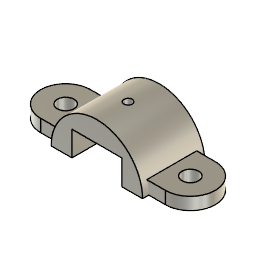
3.2 EDM (Autodesk Fusion 360 design; units mm, degrees)
Autodesk Fusion 360 part; units mm, degrees
sketch "Sketch1" plane through (0, 0, 0) normal (0, 1, 0) x (1, 0, 0)
  line L0 (-60, 0) -> (-60, -60)
  line L1 (-60, -60) -> (60, -60)
  line L2 (60, -60) -> (60, 0)
  line L3 (60, 60) -> (-60, -60) construction
  line L4 (-60, 60) -> (60, -60) construction
  arc A0 (-110, 0) -> (110, 0) centre (0, 0) ccw
  line L5 (-110, 0) -> (-60, 0)
  line L6 (60, 0) -> (110, 0)
  dimension "d1" = 220
  dimension "d2" = 120
  dimension "d3" = 120
  constraint coincident A0.centre origin
  constraint horizontal L5
  constraint parallel L0 L2
  constraint coincident L3 A0.centre
  constraint coincident L4 A0.centre
  constraint coincident L2.end L5
  constraint collinear L5 L6
  measures "d1" diameter of A0
  measures "d2" distance of L0.end L1.end
  measures "d3" distance of L4.start L0.end
extrude "Extrude1" add sketch "Sketch1" along normal mid plane 150 makes body 1
sketch "Sketch2" plane through (0, 0, 0) normal (0, 0, 1) x (1, 0, 0)
  circle A0 centre (0, 0) radius 10
  dimension "d6" = 20
  constraint coincident A0.centre origin
  measures "d6" diameter of A0
extrude "Extrude2" cut sketch "Sketch2" along normal blind 140 bodies 1
sketch "Sketch3" plane through (0, 0, 0) normal (0, 0, 1) x (1, 0, 0)
  line L0 (0, 0) -> (-153.6807, 0)
  line L1 (-153.6807, 0) -> (150, 0)
  line L2 (0, 120) -> (0, -100)
  circle A0 centre (150, 0) radius 20
  line L3 (150, 60) -> (105, 60)
  line L4 (105, 60) -> (105, 76.2902)
  line L5 (150, -60) -> (105, -60)
  line L6 (105, -60) -> (105, -75.5566)
  arc A1 (150, -60) -> (150, 60) centre (150, 0) ccw
  line L7 (105, 60) -> (105, -60)
  dimension "d9" = 120
  dimension "d10" = 40
  dimension "d11" = 150
  constraint coincident L0.start origin
  constraint horizontal L0
  constraint parallel L0 L1
  constraint perpendicular L1 L2
  constraint coincident L1.end A0.centre
  constraint concentric A0 A1
  constraint tangent L3 A1
  constraint horizontal L3
  constraint perpendicular L3 L4
  constraint tangent L5 A1
  constraint horizontal L5
  constraint perpendicular L5 L6
  constraint perpendicular L5 L7
  measures "d9" diameter of A1
  measures "d10" diameter of A0
  measures "d11" distance of L0.start L1.end
extrude "Extrude3" add sketch "Sketch3" along normal blind 30 separate body makes body 2
mirror "Mirror1" about plane through (0, 0, 0) normal (1, 0, 0) of "Extrude3" makes body 3
equation "d4 = ( 150 / 2 ) * 1 mm"
